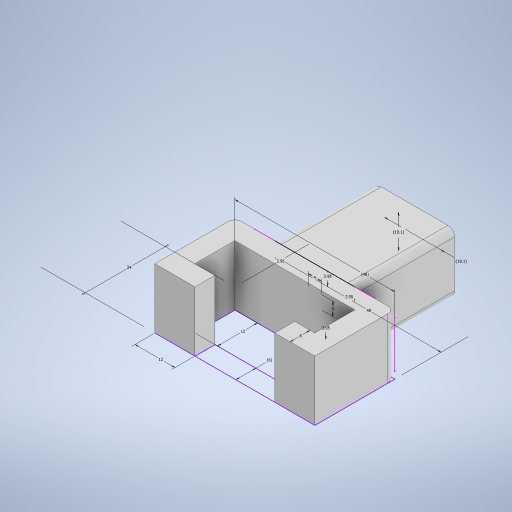
# Autodesk Inventor part: 막대꼽게1
Saved by Autodesk Inventor 2023 (Build 270158000, 158)
## iProperties
Created: 2023-04-26
Part Number: 막대꼽게1
Material: 일반
Document SubType Name: Modeling
Designer: rlatk
Density: 1 g/cm^3
Appearance: 기본값
Author: rlatk
Autodesk Inventor part; units mm, degrees
ref_plane "YZ Plane" through (0, 0, 0) normal (1, 0, 0) x (0, 1, 0)
ref_plane "XZ Plane" through (0, 0, 0) normal (0, 1, 0) x (-1, 0, 0)
ref_plane "XY Plane" through (0, 0, 0) normal (0, 0, 1) x (1, 0, 0)
sketch "스케치1" plane through (0, 0, 0) normal (0, 1, 0) x (-1, 0, 0)
  line L0 (-3.0157, 10.7069) -> (32.9843, 10.7069)
  line L1 (44.9843, 10.7069) -> (44.9843, -13.2931)
  line L2 (-3.0157, -13.2931) -> (-3.0157, 10.7069)
  line L3 (2.9843, -7.2931) -> (38.9843, -7.2931)
  line L4 (38.9843, -7.2931) -> (38.9843, 4.7069)
  line L5 (38.9843, 4.7069) -> (2.9843, 4.7069)
  line L6 (2.9843, 4.7069) -> (2.9843, -7.2931)
  line L7 (32.9843, 4.7069) -> (32.9843, 10.7069)
  line L8 (8.9843, 4.7069) -> (8.9843, 10.7069)
  line L9 (44.9843, -13.2931) -> (38.9843, -13.2931)
  line L10 (8.9843, -13.2931) -> (-3.0157, -13.2931)
  line L11 (38.9843, -13.2931) -> (8.9843, -13.2931)
  line L12 (44.9843, 10.7069) -> (32.9843, 10.7069)
  point P0 (0, 0)
  point P1 (32.9843, 7.7069)
  point P2 (8.9843, 7.7069)
  dimension "d0" = 48
  dimension "d1" = 24
  dimension "d85" = 6
  dimension "d86" = 12
  dimension "d87" = 6
  dimension "d88" = 12
  constraints: 26 end point, 5 parallel, 5 perpendicular, 5 point on line, 2 horizontal, 2 midpoint
  measures "d0" distance of L1.end L2.start
  measures "d1" distance of L1.start L1.end
  measures "d85" distance between parallel lines of L3 L11
  measures "d86" distance between parallel lines of L3 L5
  measures "d87" distance between parallel lines of L5 L0
  measures "d88" distance between parallel lines of L7 L1
ref_plane "작업 평면7" through (3.0157, 2, -13.2931) normal (0, 0, -1) x (-1, 0, 0)
sketch "스케치12" plane through (3.0157, 2, -13.2931) normal (0, 0, -1) x (-1, 0, 0)
  line L0 (0, 0) -> (0, 14) projected
  line L1 (48, 0) -> (48, 14) projected
  line L2 (42, -2) -> (6, -2) projected
  line L3 (42, 16) -> (6, 16) projected
  line L4 (36, -2) -> (36, 16) projected
  line L5 (36, -2) -> (36, 16)
  line L6 (12, -2) -> (12, 16) projected
  line L7 (12, -2) -> (12, 16)
  line L8 (36, -2) -> (12, -2)
  line L9 (12, 16) -> (36, 16)
  line L10 (0, -2) -> (48, -2) projected
  line L11 (26, 5) -> (22, 5)
  line L12 (22, 5) -> (22, 9)
  line L13 (22, 9) -> (26, 9)
  line L14 (26, 9) -> (26, 5)
  line L15 (14.95, 12.05) -> (14.95, 1.95)
  line L16 (14.95, 1.95) -> (33.05, 1.95)
  line L17 (33.05, 1.95) -> (33.05, 12.05)
  line L18 (33.05, 12.05) -> (14.95, 12.05)
  line L19 (24, 16) -> (24, 0)
  point P0 (3.0157, -2)
  point P1 (48, 7)
  point P2 (24, 5)
  dimension "d62" = 48
  dimension "d71" = 4
  dimension "d72" = 4
  dimension "d93" = 2.95
  dimension "d94" = 2.95
  dimension "d95" = 3.95
  dimension "d96" = 3.95
  constraints: 26 end point, 3 midpoint, 3 perpendicular, 2 collinear, 2 parallel, 1 horizontal, 1 point on line, 1 vertical
  measures "d62" distance from line of L0 point (48, 7)
  measures "d71" distance of L12.end L13.end
  measures "d72" distance of L11.end L12.end
  measures "d93" distance between parallel lines of L4 L17
  measures "d94" distance between parallel lines of L15 L6
  measures "d95" distance between parallel lines of L8 L16
  measures "d96" distance between parallel lines of L9 L18
extrude "돌출11" add sketch "스케치12" along normal blind 30 contours L2 L6 L3 L4 | L14 L13 L19 L18 L17 L16 L11 | L11 L19 L13 L14 | L19 L16 L15 L18 L13 L12 L11 | L11 L12 L13 L19
extrude "돌출12" cut sketch "스케치12" against normal blind 30 contours L11 L19 L13 L14 | L11 L12 L13 L19
fillet "모깎기7" radius 2 4 edges at (-8.9843, 18, -28.2931) (-32.9843, 18, -28.2931) (-32.9843, 0, -28.2931) (-8.9843, 0, -28.2931)
extrude "돌출13" cut sketch "스케치12" along normal blind 30 contours L14 L13 L19 L18 L17 L16 L11 | L19 L16 L15 L18 L13 L12 L11
extrude "돌출14" cut sketch "스케치12" along normal blind 30 contours L11 L19 L13 L14 | L11 L12 L13 L19
extrude "돌출15" add sketch "스케치1" along normal blind 18 contours L0 L8 L5 L6 L3 L4 L7 L12 L1 L9 L11 L10 L2
fillet "모깎기8" radius 2 6 edges at (-30.0343, 3.95, -28.2931) (-11.9343, 3.95, -28.2931) (-11.9343, 14.05, -28.2931) (-30.0343, 14.05, -28.2931) (3.0157, 9, -13.2931) (-44.9843, 9, -13.2931)
sketch "스케치13" plane through (-30.9843, 0, -43.2931) normal (0, -1, 0) x (1, 0, 0)
  point P0 (30.9843, 43.2931)
sketch "스케치14" plane through (3.0157, 2, -43.2931) normal (0, 0, -1) x (-1, 0, 0)
  line L0 (16.95, 12.05) -> (31.05, 12.05) projected
  line L1 (31.05, 1.95) -> (16.95, 1.95) projected
  line L2 (14.95, 3.95) -> (14.95, 10.05) projected
  line L3 (33.05, 10.05) -> (33.05, 3.95) projected
  point P0 (3.0157, -2)
  dimension "d90" = 10.1
  dimension "d91" = 18.1
  measures "d90" distance between parallel lines of L0 L1
  measures "d91" distance between parallel lines of L2 L3
